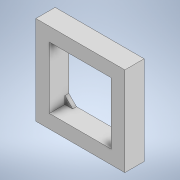
# Autodesk Inventor part: Cherry_Switch_Alignment_Jig
Saved by Autodesk Inventor 2022.2 (Build 262287000, 287)
## iProperties
Created: 2022-12-30
Part Number: Cherry_Switch_Alignment_Jig
Material: Generisch
Document SubType Name: Modeling
Designer: Frederik
Density: 1 g/cm^3
Appearance: Vorgabe
Author: Frederik
Autodesk Inventor part; units mm, degrees
ref_plane "YZ Plane" through (0, 0, 0) normal (1, 0, 0) x (0, 1, 0)
ref_plane "XZ Plane" through (0, 0, 0) normal (0, 1, 0) x (-1, 0, 0)
ref_plane "XY Plane" through (0, 0, 0) normal (0, 0, 1) x (1, 0, 0)
sketch "Skizze1" plane through (0, 0, 0) normal (0, 0, 1) x (1, 0, 0)
  line L0 (0, 0) -> (15.6, 0) construction
  line L1 (15.6, 0) -> (15.6, 15.6) construction
  line L2 (15.6, 15.6) -> (0, 15.6) construction
  line L3 (0, 15.6) -> (0, 0) construction
  line L4 (-0.2, 15.8) -> (15.8, 15.8)
  line L5 (15.8, 15.8) -> (15.8, -0.2)
  line L6 (15.8, -0.2) -> (-0.2, -0.2)
  line L7 (-0.2, -0.2) -> (-0.2, 15.8)
  line L8 (1.8, 15.8) -> (-0.2, 13.8)
  line L9 (13.8, 15.8) -> (15.8, 13.8)
  line L10 (15.8, 1.8) -> (13.8, -0.2)
  line L11 (1.8, -0.2) -> (-0.2, 1.8)
  line L12 (-0.2, -0.2) -> (15.8, 15.8) construction
  line L13 (15.8, -0.2) -> (-0.2, 15.8) construction
  line L14 (-1.725, 17.325) -> (17.325, 17.325)
  line L15 (17.325, 17.325) -> (17.325, -1.725)
  line L16 (17.325, -1.725) -> (-1.725, -1.725)
  line L17 (-1.725, -1.725) -> (-1.725, 17.325)
  point P0 (7.8, 7.8)
  point P1 (7.8, 7.8)
  dimension "d0" = 15.6
  dimension "d1" = 15.6
  dimension "d2" = 0.2
  dimension "d3" = 2
  dimension "d4" = 2
  dimension "d5" = 2
  dimension "d6" = 2
  dimension "d7" = 2
  dimension "d8" = 2
  dimension "d9" = 2
  dimension "d10" = 2
  dimension "d11" = 9.525
  constraints: 36 end point, 9 point on line, 6 parallel, 4 perpendicular, 2 midpoint, 1 horizontal, 6 other
  measures "d0" distance of L1.end L2.end
  measures "d1" distance of L0.end L1.end
  measures "d2" distance between parallel lines of L2 L4
  measures "d3" distance from line of L7 L8.start
  measures "d4" distance from line of L4 L8.end
  measures "d5" distance from line of L5 L9.start
  measures "d6" distance from line of L4 L9.end
  measures "d7" distance from line of L6 L10.start
  measures "d8" distance from line of L5 L10.end
  measures "d9" distance from line of L6 L11.end
  measures "d10" distance from line of L7 L11.start
  measures "d11" distance from line of L17 point (7.8, 7.8)
extrude "Extrusion1" add sketch "Skizze1" along normal blind 1 contours L4 L8 L7 | L4 L5 L9 | L11 L6 L7 | L5 L6 L10 | L14 L15 L16 L17
sketch "Skizze2" plane through (0, 0, 1) normal (0, 0, 1) x (1, 0, 0)
  line L0 (-1.725, -1.725) -> (17.325, -1.725) projected
  line L1 (17.325, -1.725) -> (17.325, 17.325) projected
  line L2 (17.325, 17.325) -> (-1.725, 17.325) projected
  line L3 (-1.725, 17.325) -> (-1.725, -1.725) projected
  line L4 (-0.2, 13.8) -> (1.8, 15.8) projected
  line L5 (1.8, 15.8) -> (13.8, 15.8) projected
  line L6 (13.8, 15.8) -> (15.8, 13.8) projected
  line L7 (15.8, 13.8) -> (15.8, 1.8) projected
  line L8 (15.8, 1.8) -> (13.8, -0.2) projected
  line L9 (13.8, -0.2) -> (1.8, -0.2) projected
  line L10 (1.8, -0.2) -> (-0.2, 1.8) projected
  line L11 (-0.2, 1.8) -> (-0.2, 13.8) projected
  line L12 (1.8, 15.8) -> (13.8, 15.8) projected
  line L13 (1.8, 15.8) -> (-0.2, 15.8)
  line L14 (-0.2, 15.8) -> (-0.2, 13.8)
  line L15 (-0.2, 1.8) -> (-0.2, 13.8) projected
  line L16 (-0.2, 1.8) -> (-0.2, -0.2)
  line L17 (-0.2, -0.2) -> (1.8, -0.2)
  line L18 (13.8, -0.2) -> (1.8, -0.2) projected
  line L19 (13.8, -0.2) -> (15.8, -0.2)
  line L20 (15.8, 1.8) -> (13.8, -0.2) projected
  line L21 (15.8, -0.2) -> (15.8, 1.8)
  line L22 (15.8, 13.8) -> (15.8, 1.8) projected
  line L23 (15.8, 13.8) -> (15.8, 15.8)
  line L24 (13.8, 15.8) -> (15.8, 13.8) projected
  line L25 (15.8, 15.8) -> (13.8, 15.8)
  point P0 (0, 0)
  constraints: 16 end point, 3 perpendicular, 3 point on line, 1 collinear, 1 vertical
extrude "Extrusion2" add sketch "Skizze2" along normal blind 4
pattern_of_one "Rechteckige Anordnung1"
sketch "Skizze3" plane through (0, 0, 5) normal (0, 0, 1) x (1, 0, 0)
  line L0 (17.325, -1.725) -> (17.325, 17.325) projected
  line L1 (17.325, 17.325) -> (-1.725, 17.325) projected
  line L2 (-1.725, 17.325) -> (-1.725, -1.725) projected
  line L3 (-1.725, -1.725) -> (17.325, -1.725) projected
  line L4 (-0.2, 15.8) -> (15.8, 15.8) projected
  line L5 (15.8, 15.8) -> (15.8, -0.2) projected
  line L6 (15.8, -0.2) -> (-0.2, -0.2) projected
  line L7 (-0.2, -0.2) -> (-0.2, 15.8) projected
  line L8 (-3.725, 19.325) -> (19.325, 19.325)
  line L9 (19.325, 19.325) -> (19.325, -3.725)
  line L10 (19.325, -3.725) -> (-3.725, -3.725)
  line L11 (-3.725, -3.725) -> (-3.725, 19.325)
  point P0 (0, 0)
  dimension "d22" = 2
  constraints: 8 end point, 3 other
  measures "d22" distance between parallel lines of L1 L8
extrude "Extrusion3" add sketch "Skizze3" against normal up to surface (5 mm away) contours L8 L9 L10 L11
equation "\"d1\" = d0"
equation "\"d2\" = clearance"
equation "\"d3\" = dLength"
equation "\"d4\" = dLength"
equation "\"d5\" = dLength"
equation "\"d6\" = dLength"
equation "\"d7\" = dLength"
equation "\"d8\" = dLength"
equation "\"d9\" = dLength"
equation "\"d10\" = dLength"
equation "\"d22\" = border"
equation "\"clearance\" = 0.2"
equation "\"dLength\" = 2"
equation "\"border\" = 2"
